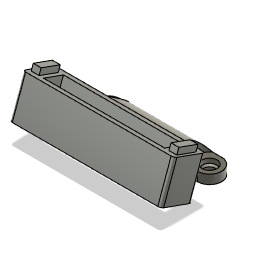
holder (Autodesk Fusion 360 design; units mm, degrees)
Autodesk Fusion 360 part; units mm, degrees
sketch "Sketch1" plane through (0, 0, 0) normal (0, 1, 0) x (1, 0, 0)
  line L0 (0, 0) -> (33.5, 0)
  circle A0 centre (0, 0) radius 1.75
  circle A1 centre (33.5, 0) radius 1.75
  circle A2 centre (33.5, 0) radius 4
  circle A3 centre (0, 0) radius 4
  line L1 (0, 4) -> (33.5, 4)
  line L2 (33.5, -4) -> (0, -4)
  dimension "d1" = 33.5
  dimension "d2" = 3.5
  dimension "d3" = 3.5
  dimension "d4" = 8
  dimension "d5" = 8
  constraint coincident L0.start A0.centre
  constraint horizontal L0
  constraint coincident L0.end A1.centre
  constraint concentric A1 A2
  constraint coincident A3 L1.start
  constraint coincident A2 L1.end
  constraint tangent A2 L1
  constraint parallel L0 L1
  constraint coincident A2 L2.start
  constraint coincident A3 L2.end
  constraint tangent A3 L2
  constraint parallel L1 L2
  measures "d1" distance of L0.start L0.end
  measures "d2" diameter of A0
  measures "d3" diameter of A1
  measures "d4" diameter of A2
  measures "d5" diameter of A3
extrude "Extrude1" add sketch "Sketch1" along normal blind 3
hole "Hole1" at (0, 3, 0) direction (0, -1, 0) diameter 5 depth 1.5 tip angle 118
hole "Hole2" at (33.5, 3, 0) direction (0, -1, 0) diameter 5 depth 1.5 tip angle 118
sketch "Sketch2" plane through (0, 3, 0) normal (0, 1, 0) x (-1, 0, 0)
  circle A0 centre (-33.5, 0) radius 2.5
  circle A1 centre (0, 0) radius 2.5
  arc A2 (0, -4) -> (0, 4) centre (0, 0) ccw
  line L0 (0, 4) -> (-33.5, 4)
  arc A3 (-33.5, 4) -> (-33.5, -4) centre (-33.5, 0) ccw
  line L1 (-33.5, -4) -> (0, -4)
  circle A4 centre (0, 0) radius 5
  circle A5 centre (-33.5, 0) radius 5
  dimension "d16" = 10
  dimension "d17" = 10
  constraint coincident A1.centre A2.centre
  constraint concentric A0 A5
  measures "d16" diameter of A4
  measures "d17" diameter of A5
extrude "Extrude2" add sketch "Sketch2" along normal blind 10 contours L0 L1 A4 A5
sketch "Sketch3" plane through (0, 0, 0) normal (1, 0, 0) x (0, 0, -1)
  line L0 (0, 0) -> (0, 3)
  line L1 (0, 3) -> (4, 3)
  line L2 (0, 3) -> (-4, 3)
  line L3 (-4, 3) -> (-4, 13)
  arc A0 (4, 3) -> (-4, 13) centre (-6.0817, 3.1346) ccw
  line L4 (-4, 13) -> (4, 13)
  line L5 (4, 13) -> (4, 3)
  dimension "d20" = 3
  dimension "d21" = 4
  dimension "d22" = 4
  dimension "d23" = 10
  dimension "d24" = 8
  constraint coincident L0.start origin
  constraint vertical L0
  constraint perpendicular L0 L1
  constraint perpendicular L0 L2
  constraint perpendicular L2 L3
  constraint perpendicular L3 L4
  measures "d20" distance of L0.start L0.end
  measures "d21" distance of L0.end L1.end
  measures "d22" distance of L0.end L2.end
  measures "d23" distance of L2.end L3.end
  measures "d24" distance of L3.end L4.end
extrude "Extrude3" cut sketch "Sketch3" along normal blind 34.5 contours A0 L4 L5
sketch "Sketch4" plane through (0, 0, 4) normal (0, 0, 1) x (1, 0, 0)
  line L0 (0, 0) -> (33.5, 0)
  line L1 (33.5, 0) -> (33.5, 3)
  line L2 (33.5, 3) -> (30.5, 3)
  line L3 (30.5, 3) -> (30.5, 13)
  line L4 (30.5, 13) -> (3, 13)
  line L5 (3, 13) -> (3, 3)
  line L6 (3, 3) -> (0, 3)
  line L7 (0, 3) -> (0, 0)
  line L8 (3, 3) -> (30.5, 3)
  constraint coincident L5.end L6.start
  constraint coincident L2.end L3.start
extrude "Extrude4" add sketch "Sketch4" along normal blind 10 contours L3 L4 L5 L8
sketch "Sketch5" plane through (3, 0, 0) normal (-1, 0, 0) x (0, 0, 1)
  line L0 (4, 13) -> (4, 3)
  line L1 (4, 3) -> (14, 3)
  line L2 (14, 3) -> (14, 13)
  line L3 (14, 13) -> (4, 13)
  line L4 (0, 0) -> (0, -6)
  line L5 (0, -6) -> (15.5, -6)
  line L6 (15.5, -6) -> (15.5, -32)
  line L7 (15.5, -32) -> (30.5, -32)
  line L8 (30.5, -32) -> (15.5, -6)
  line L9 (14, 3) -> (24.3494, 6.7268)
  line L10 (24.3494, 6.7268) -> (21.639, 14.2537)
  line L11 (14, 3) -> (11.2896, 10.5269)
  line L12 (11.2896, 10.5269) -> (21.639, 14.2537)
  line L13 (14, 3) -> (-4, 3)
  arc A0 (11.2896, 10.5269) -> (-4, 3) centre (10.0878, -6.3244) ccw
  line L14 (-4, 3) -> (-4.7957, 3)
  line L15 (-4.7957, 3) -> (-4.7957, 13)
  line L16 (-4.7957, 13) -> (4, 13)
  dimension "d29" = 6
  dimension "d30" = 15.5
  dimension "d31" = 26
  dimension "d32" = 15
  dimension "d35" = 11
  dimension "d36" = 8
  dimension "d37" = 8
  dimension "d38" = 18
  constraint coincident L4.start origin
  constraint vertical L4
  constraint perpendicular L4 L5
  constraint perpendicular L5 L6
  constraint perpendicular L6 L7
  constraint coincident L1.end L2.start
  constraint perpendicular L9 L10
  constraint perpendicular L9 L11
  constraint parallel L1 L13
  constraint parallel L13 L14
  constraint perpendicular L3 L15
  constraint coincident L0.start L3.end
  constraint perpendicular L0 L16
  measures "d29" distance of L4.start L4.end
  measures "d30" distance of L4.end L5.end
  measures "d31" distance of L5.end L6.end
  measures "d32" distance of L6.end L7.end
  measures "d35" distance of L1.end L9.end
  measures "d36" distance of L9.end L10.end
  measures "d37" distance of L1.end L11.end
  measures "d38" distance of L1.end L13.end
extrude "Extrude5" cut sketch "Sketch5" against normal blind 32 contours L0 L2 L3 L12 A0 | L0 A0 L14 L15 L16
extrude "Extrude6" cut sketch "Sketch5" against normal blind 33 contours L2 L11 L12 | L2 L9 L10 L12
extrude "Extrude7" add sketch "Sketch5" against normal blind 38.75 contours L2 L11 L12 | L2 L9 L10 L12
extrude "Extrude8" add sketch "Sketch5" along normal blind 11.25 contours L2 L11 L12 | L2 L9 L10 L12
sketch "Sketch6" plane through (0, -1.807, 0.6507) normal (0, -0.940858, 0.3388) x (1, 0, 0)
  line L0 (3, 14.1884) -> (30.5, 14.1884)
  line L1 (30.5, 14.1884) -> (41.75, 14.1884)
  line L2 (41.75, 14.1884) -> (41.75, 25.1884)
  line L3 (41.75, 25.1884) -> (-8.25, 25.1884)
  line L4 (-8.25, 25.1884) -> (-8.25, 14.1884)
  line L5 (-8.25, 14.1884) -> (3, 14.1884)
  line L6 (41.75, 14.1884) -> (40.75, 14.1884)
  line L7 (40.75, 14.1884) -> (40.75, 15.1884)
  line L8 (-8.25, 25.1884) -> (-7.25, 25.1884)
  line L9 (-7.25, 25.1884) -> (-7.25, 24.1884)
  line L10 (-8.25, 14.1884) -> (-7.25, 14.1884)
  line L11 (-7.25, 14.1884) -> (-7.25, 15.1884)
  arc A0 (40.75, 14.1884) -> (41.75, 15.1884) centre (40.75, 15.1884) ccw
  line L12 (41.75, 25.1884) -> (40.75, 25.1884)
  line L13 (40.75, 25.1884) -> (40.75, 24.1884)
  arc A1 (41.75, 24.1884) -> (40.75, 25.1884) centre (40.75, 24.1884) ccw
  arc A2 (-7.25, 25.1884) -> (-8.25, 24.1884) centre (-7.25, 24.1884) ccw
  arc A3 (-8.25, 15.144) -> (-7.25, 14.1874) centre (-7.25, 15.1884) ccw
  dimension "d47" = 1
  dimension "d48" = 1
  dimension "d50" = 1
  dimension "d51" = 1
  dimension "d52" = 1
  dimension "d53" = 1
  dimension "d83" = 1
  dimension "d84" = 1
  constraint coincident L1.end L2.start
  constraint perpendicular L2 L6
  constraint perpendicular L1 L7
  constraint coincident L3.end L4.start
  constraint perpendicular L4 L8
  constraint perpendicular L8 L9
  constraint coincident L4.end L5.start
  constraint perpendicular L4 L10
  constraint perpendicular L10 L11
  constraint coincident L2 A0.end
  constraint coincident L2.end L3.start
  constraint perpendicular L2 L12
  constraint perpendicular L12 L13
  constraint coincident L2 A1.start
  constraint coincident L4 A2.end
  constraint coincident L9.end A2.centre
  constraint coincident L4 A3.start
  constraint coincident L11.end A3.centre
  measures "d47" distance of L1.end L6.end
  measures "d48" distance of L6.end L7.end
  measures "d50" distance of L3.end L8.end
  measures "d51" distance of L8.end L9.end
  measures "d52" distance of L4.end L10.end
  measures "d53" distance of L10.end L11.end
  measures "d83" distance of L2.end L12.end
  measures "d84" distance of L12.end L13.end
extrude "Extrude9" cut sketch "Sketch6" against normal blind 9 contours L1 L2 L6 A0 | L4 L5 L10 A3 | L2 L3 L12 A1 | L3 L4 L8 A2
sketch "Sketch7" plane through (0, -1.807, 0.6507) normal (0, -0.940858, 0.3388) x (1, 0, 0)
  line L0 (-7.2944, 14.1884) -> (3, 14.1884)
  line L1 (3, 14.1884) -> (30.5, 14.1884)
  line L2 (30.5, 14.1884) -> (40.75, 14.1884)
  line L3 (41.75, 15.1884) -> (41.75, 24.1884)
  line L4 (40.75, 25.1884) -> (-7.25, 25.1884)
  line L5 (-8.25, 24.1884) -> (-8.25, 15.144)
  line L6 (-3.25, 16.1884) -> (36.75, 16.1884)
  line L7 (36.75, 16.1884) -> (36.75, 23.1884)
  line L8 (36.75, 23.1884) -> (-3.25, 23.1884)
  line L9 (-3.25, 23.1884) -> (-3.25, 16.1884)
  arc A0 (-7.25, 25.1884) -> (-8.25, 24.1884) centre (-7.25, 24.1884) ccw
  arc A1 (-8.25, 15.144) -> (-7.2944, 14.1884) centre (-7.25, 15.1884) ccw
  arc A2 (40.75, 14.1884) -> (41.75, 15.1884) centre (40.75, 15.1884) ccw
  arc A3 (41.75, 24.1884) -> (40.75, 25.1884) centre (40.75, 24.1884) ccw
  line L10 (41.75, 14.1884) -> (40.75, 14.1884)
  line L11 (40.75, 14.1884) -> (40.75, 16.1884)
  line L12 (-8.25, 14.1884) -> (-7.25, 14.1884)
  line L13 (-7.25, 14.1884) -> (-7.25, 16.1884)
  line L14 (-7.25, 16.1884) -> (-4.25, 16.1884)
  line L15 (-4.25, 16.1884) -> (-4.25, 23.1884)
  line L16 (-4.25, 23.1884) -> (-7.25, 23.1884)
  line L17 (-7.25, 23.1884) -> (-7.25, 16.1884)
  line L18 (40.75, 16.1884) -> (37.75, 16.1884)
  line L19 (37.75, 16.1884) -> (37.75, 23.1884)
  line L20 (37.75, 23.1884) -> (40.75, 23.1884)
  line L21 (40.75, 23.1884) -> (40.75, 16.1884)
  line L22 (-7.25, 14.1884) -> (-3.25, 14.1884)
  line L23 (-3.25, 14.1884) -> (-3.25, 16.1884)
  dimension "d58" = 40
  dimension "d59" = 7
  dimension "d85" = 1
  dimension "d86" = 2
  dimension "d87" = 1
  dimension "d88" = 2
  dimension "d89" = 3
  dimension "d90" = 7
  dimension "d91" = 3
  dimension "d92" = 7
  dimension "d93" = 4
  dimension "d94" = 2
  constraint horizontal L6
  constraint vertical L7
  constraint horizontal L8
  constraint vertical L9
  constraint perpendicular L3 L10
  constraint perpendicular L10 L11
  constraint perpendicular L5 L12
  constraint perpendicular L12 L13
  constraint horizontal L14
  constraint vertical L15
  constraint horizontal L16
  constraint vertical L17
  constraint horizontal L18
  constraint vertical L19
  constraint horizontal L20
  constraint vertical L21
  constraint perpendicular L13 L22
  constraint perpendicular L22 L23
  measures "d58" distance of L6.end L6.start
  measures "d59" distance of L8.end L6.start
  measures "d85" distance of L10.start L2.end
  measures "d86" distance of L2.end L11.end
  measures "d87" distance of L12.start L12.end
  measures "d88" distance of L12.end L13.end
  measures "d89" distance of L13.end L14.end
  measures "d90" distance of L13.end L16.end
  measures "d91" distance of L11.end L18.end
  measures "d92" distance of L11.end L20.end
  measures "d93" distance of L12.end L22.end
  measures "d94" distance of L22.end L6.start
extrude "Extrude10" cut sketch "Sketch7" against normal blind 16.5 contours L6 L7 L8 L9
extrude "Extrude11" cut sketch "Sketch7" against normal blind 4 contours L14 L15 L16 L17 | L18 L19 L20 L21
sketch "Sketch8" plane through (0, 5.7198, -2.0597) normal (0, 0.940858, -0.3388) x (-1, 0, 0)
  line L0 (3.25, 16.1884) -> (-36.75, 16.1884)
  line L1 (-36.75, 16.1884) -> (-36.75, 23.1884)
  line L2 (-36.75, 23.1884) -> (3.25, 23.1884)
  line L3 (3.25, 23.1884) -> (3.25, 16.1884)
  line L4 (8.25, 15.144) -> (8.25, 24.1884)
  line L5 (7.25, 25.1884) -> (-40.75, 25.1884)
  line L6 (-41.75, 24.1884) -> (-41.75, 15.1884)
  line L7 (-40.75, 14.1884) -> (-30.5, 14.1884)
  line L8 (-30.5, 14.1884) -> (-3, 14.1884)
  line L9 (-3, 14.1884) -> (7.2944, 14.1884)
  line L10 (-40.75, 14.1884) -> (-40.75, 16.4884)
  line L11 (-40.75, 16.4884) -> (-38.15, 16.4884)
  line L12 (-38.15, 16.4884) -> (-38.15, 23.1884)
  line L13 (-38.15, 23.1884) -> (-40.75, 23.1884)
  line L14 (-40.75, 23.1884) -> (-40.75, 16.4884)
  line L15 (7.2944, 14.1884) -> (7.2944, 16.4884)
  line L16 (7.2944, 16.4884) -> (4.6944, 16.4884)
  line L17 (4.6944, 16.4884) -> (4.6944, 23.1884)
  line L18 (4.6944, 23.1884) -> (7.2944, 23.1884)
  line L19 (7.2944, 23.1884) -> (7.2944, 16.4884)
  arc A0 (8.25, 24.1884) -> (7.25, 25.1884) centre (7.25, 24.1884) ccw
  arc A1 (-40.75, 25.1884) -> (-41.75, 24.1884) centre (-40.75, 24.1884) ccw
  arc A2 (-41.75, 15.1884) -> (-40.75, 14.1884) centre (-40.75, 15.1884) ccw
  arc A3 (7.2944, 14.1884) -> (8.25, 15.144) centre (7.25, 15.1884) ccw
  dimension "d71" = 2.3
  dimension "d72" = 2.6
  dimension "d73" = 6.7
  dimension "d74" = 2.3
  dimension "d75" = 2.6
  dimension "d76" = 6.7
  constraint coincident L7.start L10.start
  constraint perpendicular L7 L10
  constraint horizontal L11
  constraint vertical L12
  constraint horizontal L13
  constraint vertical L14
  constraint coincident L9.end L15.start
  constraint perpendicular L9 L15
  constraint horizontal L16
  constraint vertical L17
  constraint horizontal L18
  constraint vertical L19
  measures "d71" distance of L7.start L10.end
  measures "d72" distance of L10.end L11.end
  measures "d73" distance of L10.end L13.end
  measures "d74" distance of L9.end L15.end
  measures "d75" distance of L15.end L16.end
  measures "d76" distance of L15.end L18.end
extrude "Extrude12" add sketch "Sketch8" along normal blind 2 contours L11 L12 L13 L14 | L16 L17 L18 L19
extrude "Extrude13" add 2 faces at (-5.5611, 14.7011, 16.9785) (39.0167, 14.7011, 16.9785) along direction (0, 0.940858, -0.3388) blind 5
extrude "Extrude14" add 1 faces at (21.3333, 10.9786, 12.5441) along direction (0, 0.940858, -0.3388) blind 5
equation "d43 = -27.50 mm - 11.25 mm"
